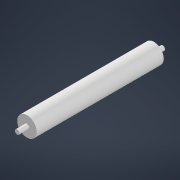
# Autodesk Inventor part: Roller
Saved by Autodesk Inventor 2021 (Build 250183000, 183)
## iProperties
Created: 2022-05-21
Part Number: Roller
Material: PET Plastic
Document SubType Name: Modeling
Designer: techv
Mass: 107.009 g
Surface Area: 344.322 cm^2
Volume: 69.4416 cm^3
Density: 1.541 g/cm^3
Appearance: Polycarbonate - Clear
Author: techv
Autodesk Inventor part; units mm, degrees
ref_plane "YZ Plane" through (0, 0, 0) normal (1, 0, 0) x (0, 1, 0)
ref_plane "XZ Plane" through (0, 0, 0) normal (0, 1, 0) x (-1, 0, 0)
ref_plane "XY Plane" through (0, 0, 0) normal (0, 0, 1) x (1, 0, 0)
sketch "Sketch1" plane through (0, 0, 0) normal (0, 0, 1) x (1, 0, 0)
  circle A0 centre (25, 25) radius 3.5 projected
  line L0 (0, 0) -> (50, 0) projected
  line L1 (50, 0) -> (50, 50) projected
  line L2 (0, 50) -> (50, 50) projected
  line L3 (0, 0) -> (0, 50) projected
extrude "Extrusion1" add sketch "Sketch1" along normal mid plane 15 contours A0
sketch "Sketch2" plane through (25, 25, -7.5) normal (0, 0, -1) x (-1, 0, 0)
  circle A0 centre (0, 0) radius 15
  point P0 (25, -25)
  dimension "d2" = 30
  constraints: 1 centre point
  measures "d2" diameter of A0
extrude "Extrusion2" add sketch "Sketch2" along normal blind 195
ref_plane "Work Plane1" through (24.9309, 25, -208.6404) normal (0.0003362, 0, 0.9999999) x (0.9999999, 0, -0.0003362)
sketch "Sketch3" plane through (24.9309, 25, -208.6404) normal (0.0003362, 0, 0.9999999) x (0.9999999, 0, -0.0003362)
  line L0 (2.0076, 1.85) -> (-2.0076, 1.85) projected
  arc A0 (-2.0076, 1.85) -> (-2.0076, -1.85) centre (0, 0) ccw projected
  line L1 (-2.0076, -1.85) -> (2.0076, -1.85) projected
  arc A1 (2.0076, -1.85) -> (2.0076, 1.85) centre (0, 0) ccw projected
  circle A2 centre (0, 0) radius 1.18 projected
  ellipse E0 centre (0, 0) end of major axis (0, 3.5) minor radius 3.5 projected
  point P0 (-25.001, -25)
extrude "Extrusion3" add sketch "Sketch3" along normal mid plane 15 contours E0
sketch "Sketch4" plane through (25, 25, -7.5) normal (0, 0, 1) x (1, 0, 0)
  circle A0 centre (0, 0) radius 12.5
  circle A1 centre (0, 0) radius 15 projected
  line L0 (-15, 0) -> (-12.5, 0)
  line L1 (-15, 0) -> (-14.3426, -1.1816) construction
  line L2 (-14.3426, -1.1816) -> (-12.242, -2.5268) construction
  spline S0 degree 2 poles (-15, 0) (-14.3426, -1.1816) (-12.242, -2.5268) knots 1 1 1 2 2 2
  line L3 (-15, 0) -> (-14.3426, 1.1816) construction
  line L4 (-14.3426, 1.1816) -> (-12.242, 2.5268) construction
  spline S1 degree 2 poles (-15, 0) (-14.3426, 1.1816) (-12.242, 2.5268) knots 1 1 1 2 2 2
  line L5 (-12.622, -6.9131) -> (-10.1558, -7.2876) construction
  spline S2 degree 2 poles (-13.7032, -6.101) (-12.622, -6.9131) (-10.1558, -7.2876) knots 1 1 1 2 2 2
  line L6 (-13.7032, -6.101) -> (-12.622, -6.9131) construction
  line L7 (-13.5832, -4.7543) -> (-12.2113, -2.6709) construction
  spline S3 degree 2 poles (-13.7032, -6.101) (-13.5832, -4.7543) (-12.2113, -2.6709) knots 1 1 1 2 2 2
  line L8 (-13.7032, -6.101) -> (-13.5832, -4.7543) construction
  line L9 (-8.719, -11.4492) -> (-6.3137, -10.7883) construction
  spline S4 degree 2 poles (-10.037, -11.1472) (-8.719, -11.4492) (-6.3137, -10.7883) knots 1 1 1 2 2 2
  line L10 (-10.037, -11.1472) -> (-8.719, -11.4492) construction
  line L11 (-10.4751, -9.868) -> (-10.0692, -7.4068) construction
  spline S5 degree 2 poles (-10.037, -11.1472) (-10.4751, -9.868) (-10.0692, -7.4068) knots 1 1 1 2 2 2
  line L12 (-10.037, -11.1472) -> (-10.4751, -9.868) construction
  line L13 (-3.3084, -14.0057) -> (-1.3799, -12.4236) construction
  spline S6 degree 2 poles (-4.6353, -14.2658) (-3.3084, -14.0057) (-1.3799, -12.4236) knots 1 1 1 2 2 2
  line L14 (-4.6353, -14.2658) -> (-3.3084, -14.0057) construction
  line L15 (-5.5558, -13.2755) -> (-6.1861, -10.862) construction
  spline S7 degree 2 poles (-4.6353, -14.2658) (-5.5558, -13.2755) (-6.1861, -10.862) knots 1 1 1 2 2 2
  line L16 (-4.6353, -14.2658) -> (-5.5558, -13.2755) construction
  line L17 (2.6743, -14.1405) -> (3.7926, -11.9108) construction
  spline S8 degree 2 poles (1.5679, -14.9178) (2.6743, -14.1405) (3.7926, -11.9108) knots 1 1 1 2 2 2
  line L18 (1.5679, -14.9178) -> (2.6743, -14.1405) construction
  line L19 (0.3241, -14.3875) -> (-1.2333, -12.439) construction
  spline S9 degree 2 poles (1.5679, -14.9178) (0.3241, -14.3875) (-1.2333, -12.439) knots 1 1 1 2 2 2
  line L20 (1.5679, -14.9178) -> (0.3241, -14.3875) construction
  line L21 (8.1946, -11.8303) -> (8.3092, -9.3384) construction
  spline S10 degree 2 poles (7.5, -12.9904) (8.1946, -11.8303) (8.3092, -9.3384) knots 1 1 1 2 2 2
  line L22 (7.5, -12.9904) -> (8.1946, -11.8303) construction
  line L23 (6.148, -13.0118) -> (3.9327, -11.8652) construction
  spline S11 degree 2 poles (7.5, -12.9904) (6.148, -13.0118) (3.9327, -11.8652) knots 1 1 1 2 2 2
  line L24 (7.5, -12.9904) -> (6.148, -13.0118) construction
  line L25 (12.2979, -7.4745) -> (11.3892, -5.1514) construction
  spline S12 degree 2 poles (12.1353, -8.8168) (12.2979, -7.4745) (11.3892, -5.1514) knots 1 1 1 2 2 2
  line L26 (12.1353, -8.8168) -> (12.2979, -7.4745) construction
  line L27 (10.9089, -9.3863) -> (8.4187, -9.2398) construction
  spline S13 degree 2 poles (12.1353, -8.8168) (10.9089, -9.3863) (8.4187, -9.2398) knots 1 1 1 2 2 2
  line L28 (12.1353, -8.8168) -> (10.9089, -9.3863) construction
  line L29 (14.2748, -1.8263) -> (12.4998, -0.0737) construction
  spline S14 degree 2 poles (14.6722, -3.1187) (14.2748, -1.8263) (12.4998, -0.0737) knots 1 1 1 2 2 2
  line L30 (14.6722, -3.1187) -> (14.2748, -1.8263) construction
  line L31 (13.7835, -4.1377) -> (11.4491, -5.0168) construction
  spline S15 degree 2 poles (14.6722, -3.1187) (13.7835, -4.1377) (11.4491, -5.0168) knots 1 1 1 2 2 2
  line L32 (14.6722, -3.1187) -> (13.7835, -4.1377) construction
  line L33 (13.7835, 4.1377) -> (11.4491, 5.0168) construction
  spline S16 degree 2 poles (14.6722, 3.1187) (13.7835, 4.1377) (11.4491, 5.0168) knots 1 1 1 2 2 2
  line L34 (14.6722, 3.1187) -> (13.7835, 4.1377) construction
  line L35 (14.2748, 1.8263) -> (12.4998, 0.0737) construction
  spline S17 degree 2 poles (14.6722, 3.1187) (14.2748, 1.8263) (12.4998, 0.0737) knots 1 1 1 2 2 2
  line L36 (14.6722, 3.1187) -> (14.2748, 1.8263) construction
  line L37 (10.9089, 9.3863) -> (8.4187, 9.2398) construction
  spline S18 degree 2 poles (12.1353, 8.8168) (10.9089, 9.3863) (8.4187, 9.2398) knots 1 1 1 2 2 2
  line L38 (12.1353, 8.8168) -> (10.9089, 9.3863) construction
  line L39 (12.2979, 7.4745) -> (11.3892, 5.1514) construction
  spline S19 degree 2 poles (12.1353, 8.8168) (12.2979, 7.4745) (11.3892, 5.1514) knots 1 1 1 2 2 2
  line L40 (12.1353, 8.8168) -> (12.2979, 7.4745) construction
  line L41 (6.148, 13.0118) -> (3.9327, 11.8652) construction
  spline S20 degree 2 poles (7.5, 12.9904) (6.148, 13.0118) (3.9327, 11.8652) knots 1 1 1 2 2 2
  line L42 (7.5, 12.9904) -> (6.148, 13.0118) construction
  line L43 (8.1946, 11.8303) -> (8.3092, 9.3384) construction
  spline S21 degree 2 poles (7.5, 12.9904) (8.1946, 11.8303) (8.3092, 9.3384) knots 1 1 1 2 2 2
  line L44 (7.5, 12.9904) -> (8.1946, 11.8303) construction
  line L45 (0.3241, 14.3875) -> (-1.2333, 12.439) construction
  spline S22 degree 2 poles (1.5679, 14.9178) (0.3241, 14.3875) (-1.2333, 12.439) knots 1 1 1 2 2 2
  line L46 (1.5679, 14.9178) -> (0.3241, 14.3875) construction
  line L47 (2.6743, 14.1405) -> (3.7926, 11.9108) construction
  spline S23 degree 2 poles (1.5679, 14.9178) (2.6743, 14.1405) (3.7926, 11.9108) knots 1 1 1 2 2 2
  line L48 (1.5679, 14.9178) -> (2.6743, 14.1405) construction
  line L49 (-5.5558, 13.2755) -> (-6.1861, 10.862) construction
  spline S24 degree 2 poles (-4.6353, 14.2658) (-5.5558, 13.2755) (-6.1861, 10.862) knots 1 1 1 2 2 2
  line L50 (-4.6353, 14.2658) -> (-5.5558, 13.2755) construction
  line L51 (-3.3084, 14.0057) -> (-1.3799, 12.4236) construction
  spline S25 degree 2 poles (-4.6353, 14.2658) (-3.3084, 14.0057) (-1.3799, 12.4236) knots 1 1 1 2 2 2
  line L52 (-4.6353, 14.2658) -> (-3.3084, 14.0057) construction
  line L53 (-10.4751, 9.868) -> (-10.0692, 7.4068) construction
  spline S26 degree 2 poles (-10.037, 11.1472) (-10.4751, 9.868) (-10.0692, 7.4068) knots 1 1 1 2 2 2
  line L54 (-10.037, 11.1472) -> (-10.4751, 9.868) construction
  line L55 (-8.719, 11.4492) -> (-6.3137, 10.7883) construction
  spline S27 degree 2 poles (-10.037, 11.1472) (-8.719, 11.4492) (-6.3137, 10.7883) knots 1 1 1 2 2 2
  line L56 (-10.037, 11.1472) -> (-8.719, 11.4492) construction
  line L57 (-13.5832, 4.7543) -> (-12.2113, 2.6709) construction
  spline S28 degree 2 poles (-13.7032, 6.101) (-13.5832, 4.7543) (-12.2113, 2.6709) knots 1 1 1 2 2 2
  line L58 (-13.7032, 6.101) -> (-13.5832, 4.7543) construction
  line L59 (-12.622, 6.9131) -> (-10.1558, 7.2876) construction
  spline S29 degree 2 poles (-13.7032, 6.101) (-12.622, 6.9131) (-10.1558, 7.2876) knots 1 1 1 2 2 2
  line L60 (-13.7032, 6.101) -> (-12.622, 6.9131) construction
  point P0 (-25, -25)
  point P1 (-12.2113, 2.6709)
  point P2 (-10.1558, 7.2876)
  point P3 (-10.0692, 7.4068)
  point P4 (-10.037, 11.1472)
  point P5 (-10.037, 11.1472)
  point P6 (-6.3137, 10.7883)
  point P7 (-6.1861, 10.862)
  point P8 (-4.6353, 14.2658)
  point P9 (-4.6353, 14.2658)
  point P10 (-1.3799, 12.4236)
  point P11 (-1.2333, 12.439)
  point P12 (1.5679, 14.9178)
  point P13 (1.5679, 14.9178)
  point P14 (3.7926, 11.9108)
  point P15 (3.9327, 11.8652)
  point P16 (7.5, 12.9904)
  point P17 (7.5, 12.9904)
  point P18 (8.3092, 9.3384)
  point P19 (8.4187, 9.2398)
  point P20 (12.1353, 8.8168)
  point P21 (12.1353, 8.8168)
  point P22 (11.3892, 5.1514)
  point P23 (11.4491, 5.0168)
  point P24 (14.6722, 3.1187)
  point P25 (14.6722, 3.1187)
  point P26 (12.4998, 0.0737)
  point P27 (12.4998, -0.0737)
  point P28 (14.6722, -3.1187)
  point P29 (14.6722, -3.1187)
  point P30 (11.4491, -5.0168)
  point P31 (11.3892, -5.1514)
  point P32 (8.4187, -9.2398)
  point P33 (8.3092, -9.3384)
  point P34 (7.5, -12.9904)
  point P35 (7.5, -12.9904)
  point P36 (3.9327, -11.8652)
  point P37 (3.7926, -11.9108)
  point P38 (1.5679, -14.9178)
  point P39 (1.5679, -14.9178)
  point P40 (-1.2333, -12.439)
  point P41 (-1.3799, -12.4236)
  point P42 (-4.6353, -14.2658)
  point P43 (-4.6353, -14.2658)
  point P44 (-6.1861, -10.862)
  point P45 (-6.3137, -10.7883)
  point P46 (-10.0692, -7.4068)
  point P47 (-10.1558, -7.2876)
  point P48 (-13.7032, -6.101)
  point P49 (-13.7032, -6.101)
  point P50 (-12.2113, -2.6709)
  dimension "d7" = 25
  dimension "d15" = 360
  constraints: 2 end point, 2 symmetric about line, 1 horizontal, 263 other
extrude "Extrusion4" cut sketch "Sketch4" against normal through all contours A0 S17 A1 S14 | A0 S19 A1 S16 | S15 A1 S12 A0 | S18 A0 S21 A1 | A1 S10 A0 S13 | S20 A0 S23 A1 | A1 S8 A0 S11 | S22 A0 S25 A1 | A1 S6 A0 S9 | S24 A0 S27 A1 | A1 S4 A0 S7 | S26 A0 S29 A1 | A1 S2 A0 S5 | S28 A0 S1 A1 | A1 S0 A0 S3
fillet "Fillet1" radius 1.5 1 edges at (10, 25, -105)
fillet "Fillet2" radius 1.5 2 edges at (12.758, 27.5268, -105) (12.758, 22.4732, -105)
pattern_circular "Circular Pattern1" count 15 over 360 about axis through (25, 25, 0) along (0, 0, 1) of "Fillet1"
ref_plane "Work Plane2" through (25, 25, -12.5) normal (0, 0, 1) x (1, 0, 0)
sketch "Sketch5" plane through (25, 25, -12.5) normal (0, 0, 1) x (1, 0, 0)
  circle A0 centre (0, 0) radius 9
  point P0 (-25, -25)
  dimension "d21" = 18
  constraints: 1 centre point
  measures "d21" diameter of A0
extrude "Extrusion5" cut sketch "Sketch5" against normal blind 185
body "Solid1"
